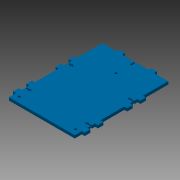
# Autodesk Inventor part: yCarPlate
Saved by Autodesk Inventor 2013 (Build 170138000, 138)
## iProperties
Created: 2015-01-14
Part Number: yCarPlate
Material: Generic
Document SubType Name: Modeling
Designer: dzban
Density: 1 g/cm^3
Author: dzban
Autodesk Inventor part; units mm, degrees
ref_plane "YZ Plane" through (0, 0, 0) normal (1, 0, 0) x (0, 1, 0)
ref_plane "XZ Plane" through (0, 0, 0) normal (0, 1, 0) x (-1, 0, 0)
ref_plane "XY Plane" through (0, 0, 0) normal (0, 0, 1) x (1, 0, 0)
sketch "Sketch1" plane through (0, 0, 0) normal (0, 0, 1) x (1, 0, 0)
  circle A0 centre (8.172, 30.7121) radius 2.4
  circle A1 centre (67.672, -114.2879) radius 2.4
  circle A2 centre (-51.328, -114.2879) radius 2.4
  line L0 (-61.328, 71.2121) -> (-61.328, 18.0121)
  line L1 (-61.328, 18.0121) -> (-67.328, 17.9121)
  line L2 (-67.328, 17.9121) -> (-67.328, 6.1121)
  line L3 (-67.328, 6.1121) -> (-61.328, 6.0121)
  line L4 (-61.328, 6.0121) -> (-61.328, -0.2879)
  line L5 (-61.328, -0.2879) -> (-54.328, -0.2879)
  line L6 (-54.328, -0.2879) -> (-54.328, 0.9621)
  line L7 (-54.328, 0.9621) -> (-52.528, 0.9621)
  line L8 (-52.528, 0.9621) -> (-52.528, -0.2879)
  line L9 (-52.528, -0.2879) -> (-49.528, -0.2879)
  line L10 (-49.528, -0.2879) -> (-49.528, -3.2879)
  line L11 (-49.528, -3.2879) -> (-52.528, -3.2879)
  line L12 (-52.528, -3.2879) -> (-52.528, -4.5379)
  line L13 (-52.528, -4.5379) -> (-54.328, -4.5379)
  line L14 (-54.328, -4.5379) -> (-54.328, -3.2879)
  line L15 (-54.328, -3.2879) -> (-61.328, -3.2879)
  line L16 (-61.328, -3.2879) -> (-61.328, -9.7879)
  line L17 (-61.328, -9.7879) -> (-67.328, -9.8879)
  line L18 (-67.328, -9.8879) -> (-67.328, -21.6879)
  line L19 (-67.328, -21.6879) -> (-61.328, -21.7879)
  line L20 (-61.328, -21.7879) -> (-61.328, -71.4879)
  line L21 (-61.328, -71.4879) -> (-67.328, -71.5879)
  line L22 (-67.328, -71.5879) -> (-67.328, -83.3879)
  line L23 (-67.328, -83.3879) -> (-61.328, -83.4879)
  line L24 (-61.328, -83.4879) -> (-61.328, -89.7879)
  line L25 (-61.328, -89.7879) -> (-54.328, -89.7879)
  line L26 (-54.328, -89.7879) -> (-54.328, -88.5379)
  line L27 (-54.328, -88.5379) -> (-52.528, -88.5379)
  line L28 (-52.528, -88.5379) -> (-52.528, -89.7879)
  line L29 (-52.528, -89.7879) -> (-49.528, -89.7879)
  line L30 (-49.528, -89.7879) -> (-49.528, -92.7879)
  line L31 (-49.528, -92.7879) -> (-52.528, -92.7879)
  line L32 (-52.528, -92.7879) -> (-52.528, -94.0379)
  line L33 (-52.528, -94.0379) -> (-54.328, -94.0379)
  line L34 (-54.328, -94.0379) -> (-54.328, -92.7879)
  line L35 (-54.328, -92.7879) -> (-61.328, -92.7879)
  line L36 (-61.328, -92.7879) -> (-61.328, -99.2879)
  line L37 (-61.328, -99.2879) -> (-67.328, -99.3879)
  line L38 (-67.328, -99.3879) -> (-67.328, -111.1879)
  line L39 (-67.328, -111.1879) -> (-61.328, -111.2879)
  line L40 (-61.328, -111.2879) -> (-61.328, -126.2879)
  line L41 (-61.328, -126.2879) -> (77.672, -126.2879)
  line L42 (77.672, -126.2879) -> (77.672, -111.2879)
  line L43 (77.672, -111.2879) -> (83.672, -111.1879)
  line L44 (83.672, -111.1879) -> (83.672, -99.3879)
  line L45 (83.672, -99.3879) -> (77.672, -99.2879)
  line L46 (77.672, -99.2879) -> (77.672, -92.9879)
  line L47 (77.672, -92.9879) -> (70.672, -92.9879)
  line L48 (70.672, -92.9879) -> (70.672, -94.2379)
  line L49 (70.672, -94.2379) -> (68.872, -94.2379)
  line L50 (68.872, -94.2379) -> (68.872, -92.9879)
  line L51 (68.872, -92.9879) -> (65.872, -92.9879)
  line L52 (65.872, -92.9879) -> (65.872, -89.9879)
  line L53 (65.872, -89.9879) -> (68.872, -89.9879)
  line L54 (68.872, -89.9879) -> (68.872, -88.7379)
  line L55 (68.872, -88.7379) -> (70.672, -88.7379)
  line L56 (70.672, -88.7379) -> (70.672, -89.9879)
  line L57 (70.672, -89.9879) -> (77.672, -89.9879)
  line L58 (77.672, -89.9879) -> (77.672, -83.4879)
  line L59 (77.672, -83.4879) -> (83.672, -83.3879)
  line L60 (83.672, -83.3879) -> (83.672, -71.5879)
  line L61 (83.672, -71.5879) -> (77.672, -71.4879)
  line L62 (77.672, -71.4879) -> (77.672, -21.6879)
  line L63 (77.672, -21.6879) -> (83.672, -21.5879)
  line L64 (83.672, -21.5879) -> (83.672, -9.7879)
  line L65 (83.672, -9.7879) -> (77.672, -9.6879)
  line L66 (77.672, -9.6879) -> (77.672, -3.3879)
  line L67 (77.672, -3.3879) -> (70.672, -3.3879)
  line L68 (70.672, -3.3879) -> (70.672, -4.6379)
  line L69 (70.672, -4.6379) -> (68.872, -4.6379)
  line L70 (68.872, -4.6379) -> (68.872, -3.3879)
  line L71 (68.872, -3.3879) -> (65.872, -3.3879)
  line L72 (65.872, -3.3879) -> (65.872, -0.3879)
  line L73 (65.872, -0.3879) -> (68.872, -0.3879)
  line L74 (68.872, -0.3879) -> (68.872, 0.8621)
  line L75 (68.872, 0.8621) -> (70.672, 0.8621)
  line L76 (70.672, 0.8621) -> (70.672, -0.3879)
  line L77 (70.672, -0.3879) -> (77.672, -0.3879)
  line L78 (77.672, -0.3879) -> (77.672, 6.1121)
  line L79 (77.672, 6.1121) -> (83.672, 6.2121)
  line L80 (83.672, 6.2121) -> (83.672, 18.0121)
  line L81 (83.672, 18.0121) -> (77.672, 18.0868)
  line L82 (77.672, 18.0868) -> (77.672, 71.1868)
  line L83 (77.672, 71.1868) -> (47.672, 71.1868)
  line L84 (47.672, 71.1868) -> (47.572, 77.1868)
  line L85 (47.572, 77.1868) -> (35.772, 77.1868)
  line L86 (35.772, 77.1868) -> (35.672, 71.1868)
  line L87 (35.672, 71.1868) -> (9.672, 71.1868)
  line L88 (9.672, 71.1868) -> (9.672, 64.1868)
  line L89 (9.672, 64.1868) -> (10.922, 64.1868)
  line L90 (10.922, 64.1868) -> (10.922, 62.3868)
  line L91 (10.922, 62.3868) -> (9.672, 62.3868)
  line L92 (9.672, 62.3868) -> (9.672, 60.9868)
  line L93 (9.672, 60.9868) -> (6.672, 60.9868)
  line L94 (6.672, 60.9868) -> (6.672, 62.3868)
  line L95 (6.672, 62.3868) -> (5.422, 62.3868)
  line L96 (5.422, 62.3868) -> (5.422, 64.1868)
  line L97 (5.422, 64.1868) -> (6.672, 64.1868)
  line L98 (6.672, 64.1868) -> (6.672, 71.1868)
  line L99 (6.672, 71.1868) -> (-19.328, 71.1868)
  line L100 (-19.328, 71.1868) -> (-19.428, 77.2121)
  line L101 (-19.428, 77.2121) -> (-31.228, 77.2121)
  line L102 (-31.228, 77.2121) -> (-31.328, 71.2121)
  line L103 (-31.328, 71.2121) -> (-61.328, 71.2121)
  point P0 (0, 0)
  point P1 (0, 0)
  constraints: 208 end point, 3 centre point
extrude "Extrusion1" add sketch "Sketch1" along normal blind 6
body "Solid1"
